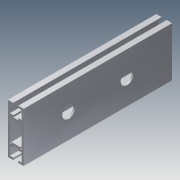
# Autodesk Inventor part: Side bar profile
Saved by Autodesk Inventor 2015 (Build 190159000, 159)
## iProperties
Created: 2016-03-14
Part Number: Side bar profile
Material: Aluminum 6061
Document SubType Name: Modeling
Designer: CretelBen
Density: 2.7 g/cm^3
Appearance: Aluminum - Flat
Author: CretelBen
Autodesk Inventor part; units mm, degrees
ref_plane "YZ Plane" through (0, 0, 0) normal (1, 0, 0) x (0, 1, 0)
ref_plane "XZ Plane" through (0, 0, 0) normal (0, 1, 0) x (-1, 0, 0)
ref_plane "XY Plane" through (0, 0, 0) normal (0, 0, 1) x (1, 0, 0)
sketch "Sketch1" plane through (0, 0, 0) normal (0, 1, 0) x (-1, 0, 0)
  line L0 (-8, 25) -> (8, 25) construction
  line L1 (8, 25) -> (8, -25)
  line L2 (8, -25) -> (-8, -25) construction
  line L3 (-8, -25) -> (-8, 25)
  line L4 (-8, 25) -> (8, -25) construction
  line L5 (8, 25) -> (-8, -25) construction
  line L6 (-8, 25) -> (-2.5, 25)
  line L7 (8, 25) -> (2.5, 25)
  line L8 (8, -25) -> (2.5, -25)
  line L9 (-8, -25) -> (-2.5, -25)
  line L10 (2.5, 25) -> (2.5, 23)
  line L11 (-2.5, 25) -> (-2.5, 23)
  line L12 (2.5, 23) -> (6, 23)
  line L13 (6, 23) -> (6, 14.25)
  line L14 (6, 14.25) -> (2.5, 14.25)
  line L15 (2.5, 14.25) -> (2.5, 12.25)
  line L16 (2.5, 12.25) -> (-2.5, 12.25)
  line L17 (-2.5, 12.25) -> (-2.5, 14.25)
  line L18 (-2.5, 14.25) -> (-6, 14.25)
  line L19 (-6, 14.25) -> (-6, 23)
  line L20 (-6, 23) -> (-2.5, 23)
  line L21 (2.5, -25) -> (2.5, -23)
  line L22 (2.5, -23) -> (6, -23)
  line L23 (6, -23) -> (6, -14.25)
  line L24 (6, -14.25) -> (2.5, -14.25)
  line L25 (2.5, -14.25) -> (2.5, -12.25)
  line L26 (2.5, -12.25) -> (-2.5, -12.25)
  line L27 (-2.5, -12.25) -> (-2.5, -14.25)
  line L28 (-2.5, -14.25) -> (-6, -14.25)
  line L29 (-6, -23) -> (-2.5, -23)
  line L30 (-2.5, -25) -> (-2.5, -23)
  line L31 (-2.5, -23) -> (-6, -23)
  line L32 (-6, -14.25) -> (-6, -23)
  line L33 (6, 12.25) -> (6, -12.25)
  line L34 (6, -12.25) -> (4.5, -12.25)
  line L35 (4.5, -12.25) -> (4.5, -10.25)
  line L36 (6, 12.25) -> (4.5, 12.25)
  line L37 (4.5, 12.25) -> (4.5, 10.25)
  line L38 (-6, 12.25) -> (-6, -12.25)
  line L39 (-6, -12.25) -> (-4.5, -12.25)
  line L40 (-4.5, -12.25) -> (-4.5, -10.25)
  line L41 (-4.5, -10.25) -> (4.5, -10.25)
  line L42 (-6, 12.25) -> (-4.5, 12.25)
  line L43 (-4.5, 12.25) -> (-4.5, 10.25)
  line L44 (-4.5, 10.25) -> (4.5, 10.25)
  point P0 (0, 0)
  dimension "d0" = 16
  dimension "d1" = 50
  dimension "d2" = 5.5
  dimension "d3" = 5.5
  dimension "d4" = 5.5
  dimension "d5" = 5.5
  dimension "d6" = 2
  dimension "d7" = 2
  dimension "d8" = 3.5
  dimension "d9" = 8.75
  dimension "d10" = 2
  dimension "d11" = 3.5
  dimension "d12" = 2
  dimension "d13" = 3.5
  dimension "d14" = 8.75
  dimension "d15" = 2
  dimension "d16" = 1.5
  dimension "d17" = 2
  dimension "d18" = 1.5
  dimension "d19" = 2
  dimension "d20" = 1.5
  dimension "d21" = 1.5
  dimension "d22" = 2
  dimension "d23" = 2
  dimension "d24" = 2
  dimension "d25" = 2
  constraints: 90 end point, 20 point on line, 19 perpendicular, 4 horizontal, 4 vertical, 3 parallel, 2 midpoint, 1 collinear
  measures "d0" distance of L1.end L2.end
  measures "d1" distance of L0.end L1.end
  measures "d2" distance of L0.start L6.end
  measures "d3" distance of L0.end L7.end
  measures "d4" distance of L1.end L8.end
  measures "d5" distance of L2.end L9.end
  measures "d6" distance of L7.end L10.end
  measures "d7" distance of L6.end L11.end
  measures "d8" distance of L10.end L12.end
  measures "d9" distance of L12.end L13.end
  measures "d10" distance of L14.end L15.end
  measures "d11" distance of L17.end L18.end
  measures "d12" distance of L8.end L21.end
  measures "d13" distance of L21.end L22.end
  measures "d14" distance of L22.end L23.end
  measures "d15" distance of L24.end L25.end
  measures "d16" distance of L33.end L34.end
  measures "d17" distance of L34.end L35.end
  measures "d18" distance of L33.start L36.end
  measures "d19" distance of L36.end L37.end
  measures "d20" distance of L38.end L39.end
  measures "d21" distance of L38.start L42.end
  measures "d22" distance between parallel lines of L1 L33
  measures "d23" distance between parallel lines of L3 L38
  measures "d24" distance between parallel lines of L14 L36
  measures "d25" distance between parallel lines of L24 L34
extrude "Extrusion1" add sketch "Sketch1" along normal blind 150
sketch "Sketch2" plane through (8, 0, 25) normal (1, 0, 0) x (0, 0, -1)
  circle A0 centre (25, 45.5) radius 6.5
  line L0 (0, 0) -> (0, 150) projected
  circle A1 centre (25, 104.5) radius 6.5
  line L1 (0, 150) -> (50, 150) projected
  point P0 (25, 0)
  dimension "d28" = 13
  dimension "d29" = 45.5
  dimension "d30" = 25
  dimension "d38" = 13
  dimension "d39" = 45.5
  dimension "d40" = 25
  constraints: 2 centre point
  measures "d28" diameter of A0
  measures "d29" distance of point (25, 0) A0.centre
  measures "d30" distance from line of A0.centre L0
  measures "d38" diameter of A1
  measures "d39" distance from line of L1 A1.centre
  measures "d40" distance from line of L0 A1.centre
hole "Hole1" at (8, 45.5, 0) at (8, 104.5, 0) direction (-1, 0, 0) diameter 13 depth 2 tip angle 118
body "Solid1"
